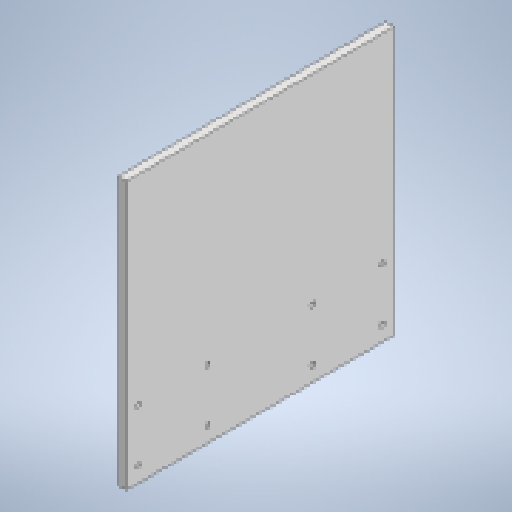
# Autodesk Inventor part: Z_PLATE
Saved by Autodesk Inventor 2023 (Build 270158000, 158)
## iProperties
Created: 2022-05-03
Part Number: Z_PLATE
Material: Generic
Document SubType Name: Modeling
Designer: plebbb
Density: 1 g/cm^3
Appearance: Default
Mass: 1048.13 g
Surface Area: 1038.64 cm^2
Volume: 1048.13 cm^3
Author: plebbb
Autodesk Inventor part; units mm, degrees
ref_plane "YZ Plane" through (0, 0, 0) normal (1, 0, 0) x (0, 1, 0)
ref_plane "XZ Plane" through (0, 0, 0) normal (0, 1, 0) x (-1, 0, 0)
ref_plane "XY Plane" through (0, 0, 0) normal (0, 0, 1) x (1, 0, 0)
sketch "Sketch1" plane through (0, 0, 0) normal (1, 0, 0) x (0, 1, 0)
  line L0 (0, 0) -> (203.2, 0)
  line L1 (203.2, 0) -> (203.2, -203.2)
  line L2 (203.2, -203.2) -> (0, -203.2)
  line L3 (0, -203.2) -> (0, 0)
  dimension "d0" = 203.2
  dimension "d1" = 203.2
  constraints: 8 end point, 2 parallel, 1 horizontal, 1 perpendicular
  measures "d0" distance of L0.end L1.end
  measures "d1" distance of L1.end L2.end
extrude "Extrusion1" add sketch "Sketch1" along normal blind 25.4
sketch "Sketch2" plane through (0, 0, 0) normal (-1, 0, 0) x (0, 0, 1)
  circle A0 centre (-141.3, 11.5) radius 2
  circle A1 centre (-141.3, 51.5) radius 2
  circle A2 centre (-194.3, 11.5) radius 2
  circle A3 centre (-194.3, 51.5) radius 2
  circle A4 centre (-8.9, 11.5) radius 2
  circle A5 centre (-8.9, 51.5) radius 2
  circle A6 centre (-61.9, 11.5) radius 2
  circle A7 centre (-61.9, 51.5) radius 2
  line L0 (-194.3, 11.5) -> (-141.3, 11.5) construction
  line L1 (-141.3, 11.5) -> (-141.3, 51.5) construction
  line L2 (-141.3, 51.5) -> (-194.3, 51.5) construction
  line L3 (-194.3, 51.5) -> (-194.3, 11.5) construction
  line L4 (-61.9, 11.5) -> (-8.9, 11.5) construction
  line L5 (-8.9, 11.5) -> (-8.9, 51.5) construction
  line L6 (-8.9, 51.5) -> (-61.9, 51.5) construction
  line L7 (-61.9, 51.5) -> (-61.9, 11.5) construction
  line L8 (0, 203.2) -> (0, 0) construction
  line L9 (-203.2, 0) -> (-203.2, 203.2) construction
  point P0 (-194.3, 31.5)
  point P1 (-8.9, 31.5)
  point P2 (0, 101.6)
  dimension "d4" = 4
  dimension "d5" = 53
  dimension "d6" = 40
  dimension "d7" = 8.9
  dimension "d8" = 8.9
  dimension "d11" = 31.5
  constraints: 16 end point, 8 centre point, 8 coincident, 7 equal radius, 4 parallel, 3 midpoint, 2 equal length, 2 horizontal, 2 perpendicular, 1 horizontal alignment
  measures "d4" diameter of A4
  measures "d5" distance of L0.start L0.end
  measures "d6" distance of L2.end L0.start
  measures "d7" distance between parallel lines of L8 L5
  measures "d8" distance from line of L9 point (-194.3, 31.5)
  measures "d11" vertical distance of L8.end point (-8.9, 31.5)
extrude "Extrusion2" cut sketch "Sketch2" against normal blind 6.35
body "Solid1"
